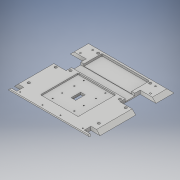
# Autodesk Inventor part: blacha
Saved by Autodesk Inventor 2019 (Build 230136000, 136)
## iProperties
Created: 2019-11-12
Part Number: blacha
Material: Generic
Document SubType Name: Modeling
Designer: Michal
Density: 1 g/cm^3
Appearance: Default
Author: Michal
Autodesk Inventor part; units mm, degrees
ref_plane "YZ Plane" through (0, 0, 0) normal (1, 0, 0) x (0, 1, 0)
ref_plane "XZ Plane" through (0, 0, 0) normal (0, 1, 0) x (-1, 0, 0)
ref_plane "XY Plane" through (0, 0, 0) normal (0, 0, 1) x (1, 0, 0)
sketch "Sketch1" plane through (0, 0, 0) normal (0, 1, 0) x (-1, 0, 0)
  line L0 (0, 0) -> (180, 0)
  line L1 (180, 0) -> (180, -180)
  line L2 (180, -180) -> (0, -180)
  line L3 (0, -180) -> (0, 0)
  line L4 (0, 0) -> (0, -4)
  line L5 (0, -4) -> (15, -4)
  line L6 (15, -4) -> (15, -19)
  line L7 (15, -19) -> (0, -19)
  line L8 (0, -19) -> (0, -4)
  line L9 (90, 0) -> (90, -180)
  line L10 (180, 0) -> (180, -4)
  line L11 (180, -4) -> (165, -4)
  line L12 (165, -4) -> (165, -19)
  line L13 (165, -19) -> (180, -19)
  line L14 (180, -19) -> (180, -4)
  dimension "d0" = 180
  dimension "d1" = 180
  dimension "d2" = 4
  dimension "d3" = 15
  dimension "d4" = 15
  constraints: 30 end point, 4 parallel, 4 symmetric about line, 2 horizontal, 2 midpoint, 2 perpendicular, 1 point on line
  measures "d0" distance of L1.end L2.end
  measures "d1" distance of L0.end L1.end
  measures "d2" distance of L0.start L4.end
  measures "d3" distance of L6.end L7.end
  measures "d4" distance of L5.end L6.end
extrude "Extrusion1" add sketch "Sketch1" along normal blind 8 contours L0 L9 L2 L3 L7 L6 L5 | L0 L1 L11 L12 L13 L2 L9
sketch "Sketch3" plane through (0, 8, 0) normal (0, 1, 0) x (1, 0, 0)
  line L0 (0, 180) -> (-180, 180) projected
  line L1 (0, 180) -> (-30, 180)
  line L2 (-30, 180) -> (-30, 96)
  line L3 (-30, 96) -> (0, 96)
  line L4 (0, 96) -> (0, 180)
  line L5 (-30, 96) -> (-30, 146)
  line L6 (-30, 146) -> (0, 146)
  line L7 (0, 19) -> (0, 180) projected
  line L8 (-30, 96) -> (0, 96)
  line L9 (0, 96) -> (0, 146)
  line L10 (-90, 180) -> (-90, 0)
  line L11 (-180, 180) -> (-150, 180)
  line L12 (-150, 180) -> (-150, 96)
  line L13 (-150, 96) -> (-180, 96)
  line L14 (-180, 96) -> (-180, 180)
  line L15 (-150, 96) -> (-150, 146)
  line L16 (-150, 146) -> (-180, 146)
  line L17 (-150, 96) -> (-180, 96)
  line L18 (-180, 96) -> (-180, 146)
  point P0 (0, 0)
  dimension "d40" = 30
  dimension "d41" = 84
  dimension "d42" = 50
  constraints: 34 end point, 5 symmetric about line, 3 perpendicular, 3 point on line, 2 parallel, 1 collinear, 1 horizontal, 1 midpoint, 1 vertical
  measures "d40" distance of L3.end L2.end
  measures "d41" distance of L2.end L1.end
  measures "d42" distance of L2.end L5.end
extrude "Extrusion2" cut sketch "Sketch3" against normal blind 8 contours L4 L3 L2 L6 | L12 L13 L14 L16
sketch "Sketch4" plane through (0, 0, 0) normal (0, -1, 0) x (1, 0, 0)
  line L0 (0, 0) -> (-180.0098, 0)
  line L1 (-180.0098, 0) -> (-180.0098, -9.1)
  line L2 (-180.0098, -9.1) -> (0, -9.1)
  line L3 (0, -9.1) -> (0, 0)
  dimension "d14" = 180.0098
  dimension "d15" = 9.1
  constraints: 8 end point, 2 parallel, 1 horizontal, 1 perpendicular
  measures "d14" distance of L2.end L1.end
  measures "d15" distance of L1.end L0.end
extrude "Extrusion3" cut sketch "Sketch4" against normal blind 5
sketch "Sketch5" plane through (0, 8, 0) normal (0, 1, 0) x (1, 0, 0)
  line L0 (-0.001, 131.5) -> (-62.0024, 131.5)
  line L1 (-0.001, 110.5) -> (-62.0024, 110.5)
  line L2 (-180.0014, 131.5) -> (-118, 131.5)
  line L3 (-180.0014, 110.5) -> (-118, 110.5)
  line L4 (-62.0024, 110.5) -> (-118, 110.5)
  line L5 (-118, 131.5) -> (-62.0024, 131.5)
  line L6 (-180.0014, 110.5) -> (-180.0014, 131.5)
  line L7 (-0.001, 131.5) -> (-0.001, 110.5)
  line L8 (-150, 146) -> (-150, 96) projected
  line L9 (-150, 150.5) -> (-150, 125.5)
  line L10 (-180.0014, 121) -> (-150, 121)
  point P0 (0, 0)
  point P1 (-61.993, 96)
  point P2 (-118, 96)
  dimension "d19" = 62.0014
  dimension "d21" = 62.0014
  dimension "d47" = 20.5
  constraints: 20 end point, 2 parallel, 1 coincident, 1 horizontal, 1 midpoint, 1 perpendicular, 1 vertical
  measures "d19" distance of L0.end L0.start
  measures "d21" distance of L1.start L1.end
  measures "d47" distance of L8.start L9.end
extrude "Extrusion4" cut sketch "Sketch5" against normal blind 5.5
sketch "Sketch8" plane through (0, 8, 0) normal (0, 1, 0) x (1, 0, 0)
  line L0 (-150, 131.5) -> (-147, 131.5)
  line L1 (-30, 131.5) -> (-33, 131.5)
  line L2 (-40, 131.5) -> (-140, 131.5)
  line L3 (-150, 131.5) -> (-30, 131.5) projected
  line L4 (-150, 131.5) -> (-30, 131.5) projected
  line L5 (-140, 131.5) -> (-137, 131.5)
  line L6 (-137, 171.5) -> (-43, 171.5)
  line L7 (-140, 131.5) -> (-143, 131.5)
  line L8 (-143, 131.5) -> (-143, 171.5)
  line L9 (-43, 131.5) -> (-37, 131.5)
  line L10 (-37, 131.5) -> (-37, 171.5)
  line L11 (-37, 171.5) -> (-143, 171.5)
  point P0 (0, 0)
  dimension "d43" = 3
  dimension "d45" = 3
  dimension "d171" = 3
  dimension "d172" = 3
  dimension "d176" = 3
  dimension "d177" = 6
  constraints: 20 end point, 2 collinear, 2 perpendicular, 5 other
  measures "d43" distance of L0.start L0.end
  measures "d45" distance of L1.start L1.end
  measures "d171" distance of L2.start L9.start
  measures "d172" distance of L2.end L5.end
  measures "d176" distance of L2.end L7.end
  measures "d177" distance of L9.start L9.end
extrude "Extrusion7" cut sketch "Sketch8" against normal blind 4.5
fillet "Fillet1" radius 2 2 edges at (-143, 5.75, -171.5) (-37, 5.75, -171.5)
sketch "Sketch9" plane through (0, 8, 0) normal (0, 1, 0) x (1, 0, 0)
  line L0 (-30, 110.5) -> (-150, 110.5) projected
  line L1 (-90, 110.5) -> (-90, 107.5)
  line L2 (-90, 107.5) -> (-130, 107.5)
  line L3 (-130, 107.5) -> (-130, 27.5)
  line L4 (-130, 27.5) -> (-50, 27.5)
  line L5 (-50, 27.5) -> (-50, 107.5)
  line L6 (-50, 107.5) -> (-90, 107.5)
  point P0 (0, 0)
  dimension "d48" = 3
  dimension "d49" = 40
  dimension "d50" = 80
  dimension "d51" = 80
  constraints: 12 end point, 3 perpendicular, 2 horizontal, 1 midpoint, 1 vertical
  measures "d48" distance of L1.start L1.end
  measures "d49" distance of L1.end L2.end
  measures "d50" distance of L2.end L3.end
  measures "d51" distance of L3.end L4.end
extrude "Extrusion8" cut sketch "Sketch9" against normal blind 3
sketch "Sketch10" plane through (0, 5, 0) normal (0, 1, 0) x (1, 0, 0)
  line L0 (-130, 107.5) -> (-50, 107.5) projected
  line L1 (-130, 107.5) -> (-114.1, 107.5)
  line L2 (-114.1, 107.5) -> (-114.1, 102.1)
  line L3 (-114.1, 102.1) -> (-114.1, 53.9)
  line L4 (-90, 107.5) -> (-90, 27.5)
  line L5 (-50, 27.5) -> (-130, 27.5) projected
  line L6 (-50, 107.5) -> (-65.9, 107.5)
  line L7 (-65.9, 107.5) -> (-65.9, 102.1)
  line L8 (-65.9, 102.1) -> (-65.9, 53.9)
  line L9 (-130, 27.5) -> (-130, 107.5) projected
  line L10 (-130, 67.5) -> (-48.2332, 67.5)
  line L11 (-130, 27.5) -> (-50, 27.5)
  line L12 (-130, 27.5) -> (-114.1, 27.5)
  line L13 (-114.1, 27.5) -> (-114.1, 32.9)
  line L14 (-114.1, 32.9) -> (-114.1, 81.1)
  line L15 (-90, 27.5) -> (-90, 107.5)
  line L16 (-50, 107.5) -> (-130, 107.5)
  line L17 (-50, 27.5) -> (-65.9, 27.5)
  line L18 (-65.9, 27.5) -> (-65.9, 32.9)
  line L19 (-65.9, 32.9) -> (-65.9, 81.1)
  line L20 (-130, 107.5) -> (-130, 27.5)
  point P0 (0, 0)
  dimension "d86" = 15.9
  dimension "d87" = 5.4
  dimension "d88" = 48.2
  constraints: 36 end point, 15 symmetric about line, 3 midpoint, 2 point on line, 2 vertical, 1 perpendicular
  measures "d86" distance of L0.start L1.end
  measures "d87" distance of L1.end L2.end
  measures "d88" distance of L2.end L3.end
move faces "Move1" translate (0, 0, 4) faces at (-103.3333, 7, -27.5)
move faces "Move2" translate (-2, 0, 0) faces at (-130, 6, -79.5)
move faces "Move3" translate (2, 0, 0) faces at (-50, 7, -51.5)
fillet "Fillet2" radius 2 4 edges at (-132, 6.5, -23.5) (-48, 6.5, -23.5) (-48, 6.5, -107.5) (-132, 6.5, -107.5)
sketch "Sketch11" plane through (0, 5, 0) normal (0, -1, 0) x (1, 0, 0)
  line L0 (-165, -9.1) -> (-165, -4) projected
  line L1 (-165, -9.1) -> (-165, -6.1)
  line L2 (-165, -6.1) -> (-160, -6.1)
  line L3 (-160, -6.1) -> (-110, -6.1)
  line L4 (-180, 0) -> (0, 0) projected
  line L5 (-90, 0) -> (-90, -9.1)
  line L6 (-15, -9.1) -> (-165, -9.1) projected
  line L7 (-15, -9.1) -> (-15, -4)
  line L8 (-15, -9.1) -> (-15, -6.1)
  line L9 (-15, -6.1) -> (-20, -6.1)
  line L10 (-20, -6.1) -> (-70, -6.1)
  line L11 (0, 0) -> (-180, 0)
  line L12 (-165, -9.1) -> (-15, -9.1)
  dimension "d64" = 3
  dimension "d65" = 5
  dimension "d66" = 50
  constraints: 20 end point, 8 symmetric about line, 4 point on line, 2 midpoint, 1 perpendicular
  measures "d64" distance of L0.start L1.end
  measures "d65" distance of L1.end L2.end
  measures "d66" distance of L2.end L3.end
hole "Hole1" at (-160, 5, -6.1) at (-110, 5, -6.1) at (-70, 5, -6.1) at (-20, 5, -6.1) direction (0, 1, 0) diameter 2.4638 end through all
move faces "Move4" translate (0, 0, 2.5) faces at (-10, 5.3333, -146)
move faces "Move5" translate (0, 0, 2.5) faces at (-160, 5.3333, -146)
move faces "Move6" translate (0, 0, -2.5) faces at (-160, 2.6667, -96)
move faces "Move7" translate (0, 0, -2.5) faces at (-20, 5.3333, -96)
hole "Hole2" at (-114.1, 5, -102.1) at (-114.1, 5, -53.9) at (-65.9, 5, -53.9) at (-65.9, 5, -102.1) at (-114.1, 5, -81.1) at (-114.1, 5, -32.9) at (-65.9, 5, -32.9) at (-65.9, 5, -81.1) direction (0, -1, 0) diameter 2.4638 end through all
sketch "Sketch15" plane through (0, 0, 0) normal (0, -1, 0) x (1, 0, 0)
  line L0 (0, -180) -> (-180, -180) projected
  line L1 (-180, 0) -> (0, 0) projected
  line L2 (-90, 0) -> (-90, -180)
  line L3 (-149.9592, -180) -> (-149.9592, -168)
  line L4 (-180, -98.5) -> (-150, -98.5)
  line L5 (-149.9592, -168) -> (-159.9592, -168)
  line L6 (-180, -143.5) -> (-150, -143.5)
  line L7 (-180, -143.5) -> (-180, -148.5)
  line L8 (-180, -143.5) -> (-180, -180)
  line L9 (-180, -148.5) -> (-168, -148.5)
  line L10 (-180, -98.5) -> (-168, -98.5)
  line L11 (-150, -98.5) -> (-180, -98.5)
  line L12 (-168, -98.5) -> (-168, -93.5)
  line L13 (-168, -93.5) -> (-168, -33.5)
  line L14 (-149.9592, -168) -> (-147.9592, -168)
  line L15 (-150, -110.5) -> (-150, -98.5) projected
  line L16 (-150, -98.5) -> (-150, -103.5)
  line L17 (-150, -103.5) -> (-145, -103.5)
  line L18 (0, -98.5) -> (-30, -98.5)
  line L19 (-30, -98.5) -> (0, -98.5)
  line L20 (-12, -98.5) -> (-12, -93.5)
  line L21 (-12, -93.5) -> (-12, -33.5)
  line L22 (0, -98.5) -> (-12, -98.5)
  line L23 (0, -143.5) -> (-30, -143.5)
  line L24 (0, -148.5) -> (-12, -148.5)
  line L25 (0, -143.5) -> (0, -148.5)
  line L26 (-30.0408, -168) -> (-20.0408, -168)
  line L27 (0, -143.5) -> (0, -180)
  line L28 (-30.0408, -180) -> (-30.0408, -168)
  line L29 (-30.0408, -168) -> (-32.0408, -168)
  line L30 (-30, -110.5) -> (-30, -98.5)
  line L31 (-30, -98.5) -> (-30, -103.5)
  line L32 (-30, -103.5) -> (-35, -103.5)
  point P0 (-165, -19)
  point P1 (-180, -19)
  point P2 (-15, -19)
  point P3 (0, -19)
  dimension "d173" = 2
  dimension "d174" = 5
  dimension "d175" = 5
  constraints: 60 end point, 18 symmetric about line, 8 point on line, 2 midpoint, 1 horizontal, 1 perpendicular
  measures "d173" distance of L5.start L14.end
  measures "d174" distance of L4.end L16.end
  measures "d175" distance of L16.end L17.end
hole "Hole3" at (-168, 0, -33.5) at (-168, 0, -93.5) at (-145, 0, -103.5) at (-147.9592, 0, -168) at (-12, 0, -33.5) at (-35, 0, -103.5) at (-32.0408, 0, -168) at (-12, 0, -93.5) direction (0, 1, 0) diameter 5.4 end through all countersink diameter 10.3886 countersink angle 90 clearance for "Countersunk Flat Head Screw ISO 2009/7046" size "M5" standard "ISO"
sketch "Sketch16" plane through (0, 0, -180) normal (1, 0, 0) x (0, 0, -1)
  line L0 (0, 0) -> (0, 8) projected
  line L1 (0, 8) -> (3, 8)
  line L2 (3, 8) -> (-11.8412, 22.8412)
  line L3 (-11.8412, 22.8412) -> (-13.9625, 20.7199)
  line L4 (-13.9625, 20.7199) -> (-1.2426, 8)
  line L5 (-36.5, 8) -> (0, 8) projected
  line L6 (0, 6.7574) -> (0, 8)
  line L7 (0, 8) -> (-1.2426, 8)
  line L8 (0, 6.7574) -> (-1.2426, 8)
  point P0 (-180, 0)
  dimension "d133" = 3
  dimension "d134" = 45
  dimension "d135" = 3
  constraints: 14 end point, 2 collinear, 2 perpendicular, 2 point on line, 1 horizontal, 1 vertical
  measures "d133" distance of L0.end L1.end
  measures "d134" angle of L2 L1
  measures "d135" distance of L2.end L3.end
extrude "Extrusion9" cut sketch "Sketch16" against normal blind 180 contours L8 L5 L0
sketch "Sketch17" plane through (-180, 8, 0) normal (0, 0, 1) x (1, 0, 0)
  line L0 (180, 0) -> (180, -8) projected
  line L1 (180, 0) -> (183, 0)
  line L2 (183, 0) -> (173.5168, 9.4832)
  line L3 (173.5168, 9.4832) -> (171.3955, 7.3618)
  line L4 (171.3955, 7.3618) -> (178.7574, 0)
  line L5 (180, 0) -> (0, 0) projected
  line L6 (178.7574, 0) -> (180, 0)
  line L7 (178.7574, 0) -> (180, -1.2426)
  line L8 (180, 0) -> (180, -1.2426)
  line L9 (180, -8) -> (0, -8) projected
  line L10 (90, -8) -> (90, 18.8619)
  line L11 (0, 0) -> (0, -8)
  line L12 (0, 0) -> (-3, 0)
  line L13 (-3, 0) -> (6.4832, 9.4832)
  line L14 (6.4832, 9.4832) -> (8.6045, 7.3618)
  line L15 (8.6045, 7.3618) -> (1.2426, 0)
  line L16 (1.2426, 0) -> (0, 0)
  line L17 (1.2426, 0) -> (0, -1.2426)
  line L18 (0, 0) -> (0, -1.2426)
  dimension "d138" = 3
  dimension "d139" = 13.4112
  dimension "d140" = 45
  dimension "d141" = 3
  constraints: 32 end point, 5 symmetric about line, 4 point on line, 2 collinear, 1 horizontal, 1 midpoint, 1 parallel, 1 perpendicular, 1 vertical
  measures "d138" distance of L0.start L1.end
  measures "d139" distance of L1.end L2.end
  measures "d140" angle of L2 L1
  measures "d141" distance of L2.end L3.end
extrude "Extrusion10" cut sketch "Sketch17" against normal blind 180 contours L0 L7 L5 | L17 L11 L5
sketch "Sketch19" plane through (0, 0, -143.5) normal (1, 0, 0) x (0, 0, -1)
  line L0 (0, 6.7574) -> (36.5, 6.7574) projected
  line L1 (36.5, 0) -> (36.5, 6.7574) projected
  line L2 (36.5, 6.7574) -> (36.5, 0)
  line L3 (36.5, 6.7574) -> (50.6986, 6.7574) construction
  line L4 (36.5, 0) -> (43.2574, 0)
  line L5 (36.5, 6.7574) -> (43.2574, 0)
  point P0 (-143.5, 0)
  constraints: 8 end point, 1 collinear, 1 horizontal, 1 perpendicular
extrude "Extrusion11" add sketch "Sketch19" against normal blind 180
sketch "Sketch20" plane through (-180, 5, 0) normal (0, 0, 1) x (1, 0, 0)
  line L0 (0, 1.7574) -> (1.2426, 3) projected
  line L1 (0, 0) -> (180, 0) projected
  line L2 (0, 1.7574) -> (0, 0)
  line L3 (0, 1.7574) -> (6.1976, 1.7574) construction
  line L4 (0, 0) -> (-1.7574, 0)
  line L5 (0, 1.7574) -> (0, -5) projected
  line L6 (-1.7574, 0) -> (0, 1.7574)
  line L7 (50, 3) -> (130, 3) projected
  line L8 (90, 3) -> (90, -5)
  line L9 (180, 1.7574) -> (178.7574, 3)
  line L10 (180, 1.7574) -> (180, 0)
  line L11 (180, 1.7574) -> (173.8024, 1.7574) construction
  line L12 (180, 0) -> (181.7574, 0)
  line L13 (180, 1.7574) -> (180, -5)
  line L14 (181.7574, 0) -> (180, 1.7574)
  constraints: 22 end point, 5 symmetric about line, 2 horizontal, 1 collinear, 1 midpoint, 1 perpendicular, 1 vertical
extrude "Extrusion12" add sketch "Sketch20" against normal blind 4
sketch "Sketch21" plane through (-15, 0, -19) normal (0, 0, 1) x (1, 0, 0)
  line L0 (15, 6.7574) -> (15, 0) projected
  line L1 (15, 6.7574) -> (15, 0)
  line L2 (15, 6.7574) -> (25.4889, -3.7316)
  line L3 (15, 6.7574) -> (29.8336, 6.7574) construction
  line L4 (15, 0) -> (21.7574, 0)
  line L5 (15, 6.7574) -> (21.7574, 0)
  line L6 (-115, 8) -> (-35, 8) projected
  line L7 (-75, 8) -> (-75, 0)
  line L8 (-165, 6.7574) -> (-165, 0)
  line L9 (-165, 6.7574) -> (-165, 0)
  line L10 (-165, 6.7574) -> (-175.4889, -3.7316)
  line L11 (-165, 6.7574) -> (-179.8336, 6.7574) construction
  line L12 (-165, 0) -> (-171.7574, 0)
  line L13 (-165, 6.7574) -> (-171.7574, 0)
  dimension "d154" = 14.8336
  dimension "d155" = 45
  constraints: 24 end point, 5 symmetric about line, 2 horizontal, 2 point on line, 2 vertical, 1 collinear, 1 equal length, 1 midpoint
  measures "d154" distance of L0.start L2.end
  measures "d155" angle of L2 L3
extrude "Extrusion13" add sketch "Sketch21" against normal blind 170
sketch "Sketch22" plane through (0, 0, -189) normal (-1, 0, 0) x (0, 0, 1)
  line L0 (10.2426, 8) -> (45.5, 8) projected
  line L1 (9, 6.7574) -> (2.2426, 0) projected
  line L2 (10.2426, 8) -> (2.2426, 0)
  line L3 (170, 0) -> (0, 0) projected
  line L4 (2.2426, 0) -> (0, 0)
  line L5 (0, 6.7574) -> (0, 0) projected
  line L6 (0, 0) -> (0, 6.7574)
  line L7 (0, 6.7574) -> (10.2426, 8)
  point P0 (189, 0)
  constraints: 8 end point, 3 collinear
extrude "Extrusion14" cut sketch "Sketch22" along normal mid plane 762
sketch "Sketch23" plane through (0, 8, 0) normal (0, 1, 0) x (1, 0, 0)
  line L0 (-180, 98.5) -> (-180, 143.5) projected
  line L1 (-180, 143.5) -> (-180, 98.5)
  line L2 (-180, 98.5) -> (-186.7574, 98.5)
  line L3 (-186.7574, 19) -> (-186.7574, 186.7574) projected
  line L4 (-186.7574, 143.5) -> (-180, 143.5)
  line L5 (-186.7574, 143.5) -> (-186.7574, 98.5)
  line L6 (0, 98.5) -> (0, 143.5) projected
  line L7 (0, 143.5) -> (6.7574, 143.5)
  line L8 (6.7574, 19) -> (6.7574, 186.7574) projected
  line L9 (6.7574, 98.5) -> (6.7574, 143.5)
  line L10 (6.7574, 98.5) -> (0, 98.5)
  line L11 (0, 98.5) -> (0, 143.5)
  point P0 (0, 0)
  constraints: 16 end point, 4 point on line, 3 collinear, 2 horizontal, 2 perpendicular, 1 parallel
extrude "Extrusion15" cut sketch "Sketch23" against normal blind 762
sketch "Sketch24" plane through (-181.7574, 5, 0) normal (0, 0, 1) x (1, 0, 0)
  line L0 (180.5147, 3) -> (3, 3) projected
  line L1 (180.5147, 3) -> (179.0147, 3)
  line L2 (-5, -5) -> (188.5147, -5) projected
  line L3 (188.5147, -5) -> (187.0147, -5)
  line L4 (187.0147, -5) -> (179.0147, 3)
  line L5 (180.5147, 3) -> (188.5147, -5)
  line L6 (151.7574, 3) -> (31.7574, 3) projected
  line L7 (91.7574, 3) -> (91.7574, -5)
  line L8 (3, 3) -> (4.5, 3)
  line L9 (-5, -5) -> (-3.5, -5)
  line L10 (-3.5, -5) -> (4.5, 3)
  line L11 (3, 3) -> (-5, -5)
  point P0 (181.7574, -5)
  point P1 (1.7574, -5)
  dimension "d162" = 1.5
  dimension "d163" = 1.5
  constraints: 18 end point, 3 point on line, 3 symmetric about line, 1 midpoint, 1 perpendicular
  measures "d162" distance of L0.start L1.end
  measures "d163" distance of L2.end L3.end
extrude "Extrusion16" cut sketch "Sketch24" against normal blind 200 contours L5 L2 L4 L0 | L2 L11 L0 L10
sketch "Sketch25" plane through (-30, 2.5, -131.5) normal (1, 0, 0) x (0, 0, -1)
  line L0 (47.2574, 5.5) -> (45.2574, 5.5)
  line L1 (12, 5.5) -> (47.2574, 5.5) projected
  line L2 (55.2574, -2.5) -> (12, -2.5) projected
  line L3 (55.2574, -2.5) -> (53.2574, -2.5)
  line L4 (53.2574, -2.5) -> (45.2574, 5.5)
  line L5 (47.2574, 5.5) -> (55.2574, -2.5)
  line L6 (45.2574, 5.5) -> (44.2574, 5.5)
  line L7 (44.2574, 5.5) -> (52.2574, -2.5)
  line L8 (53.2574, -2.5) -> (52.2574, -2.5)
  point P0 (-131.5, -2.5)
  dimension "d166" = 2
  dimension "d167" = 2
  dimension "d170" = 1
  constraints: 14 end point, 4 point on line, 1 parallel
  measures "d166" distance of L0.start L0.end
  measures "d167" distance of L2.start L3.end
  measures "d170" distance of L0.end L6.end
extrude "Extrusion17" cut sketch "Sketch25" along normal mid plane 1016
sketch "Sketch26" plane through (0, 0, 0) normal (0, -1, 0) x (1, 0, 0)
  line L0 (-177.2574, 0) -> (-2.7426, 0) construction
  line L1 (-90, 0) -> (-90, -183.7574) construction
  line L2 (-185.2574, -183.7574) -> (5.2574, -183.7574) construction
  line L3 (-150, -143.5) -> (-185.2574, -143.5) construction
  point P0 (0, 0)
  point P1 (-168, -148.5)
  point P2 (-160, -168)
  point P3 (-12, -148.5)
  point P4 (-20, -168)
  dimension "d199" = 78
  dimension "d200" = 5
  dimension "d201" = 70
  dimension "d202" = 24.5
  constraints: 2 end point, 2 midpoint, 2 symmetric about line
  measures "d199" distance from line of L1 point (-168, -148.5)
  measures "d200" distance from line of L3 point (-168, -148.5)
  measures "d201" distance from line of L1 point (-160, -168)
  measures "d202" distance from line of L3 point (-160, -168)
hole "Hole4" at (-20, 0, -168) at (-12, 0, -148.5) at (-168, 0, -148.5) at (-160, 0, -168) direction (0, 1, 0) diameter 3.4 end through all countersink diameter 6.9 countersink angle 81.933 clearance for "Countersunk Flat Head Screw ISO 2009/7046" size "M3" standard "ISO"
sketch "Sketch27" plane through (0, 5, 0) normal (0, 1, 0) x (1, 0, 0)
  line L0 (-50, 23.5) -> (-130, 23.5) projected
  line L1 (-90, 23.5) -> (-90, 107.5)
  line L2 (-130, 107.5) -> (-50, 107.5) projected
  circle A0 centre (-114.1, 53.9) radius 1.2319 projected
  line L3 (-114.1, 53.9) -> (-95.1, 53.9)
  line L4 (-95.1, 53.9) -> (-95.1, 55.9)
  line L5 (-95.1, 55.9) -> (-95.1, 62.9)
  circle A1 centre (-65.9, 53.9) radius 1.2319
  line L6 (-65.9, 53.9) -> (-84.9, 53.9)
  line L7 (-84.9, 53.9) -> (-84.9, 55.9)
  line L8 (-84.9, 55.9) -> (-84.9, 62.9)
  line L9 (-84.9, 62.9) -> (-95.1, 62.9)
  line L10 (-95.1, 53.9) -> (-84.9, 53.9)
  line L11 (-132, 25.5) -> (-132, 105.5) projected
  line L12 (-132, 65.5) -> (-48.3182, 65.5)
  circle A2 centre (-114.1, 77.1) radius 1.2319
  line L13 (-114.1, 77.1) -> (-95.1, 77.1)
  line L14 (-95.1, 77.1) -> (-95.1, 75.1)
  line L15 (-95.1, 75.1) -> (-95.1, 68.1)
  circle A3 centre (-65.9, 77.1) radius 1.2319
  line L16 (-65.9, 77.1) -> (-84.9, 77.1)
  line L17 (-84.9, 77.1) -> (-84.9, 75.1)
  line L18 (-84.9, 75.1) -> (-84.9, 68.1)
  line L19 (-84.9, 68.1) -> (-95.1, 68.1)
  line L20 (-95.1, 77.1) -> (-84.9, 77.1)
  point P0 (0, 0)
  dimension "d185" = 19
  dimension "d186" = 2
  dimension "d187" = 7
  constraints: 36 end point, 12 symmetric about line, 4 point on line, 3 centre point, 3 midpoint, 3 perpendicular, 1 collinear, 1 horizontal, 3 other
  measures "d185" distance of L3.start L3.end
  measures "d186" distance of L3.end L4.end
  measures "d187" distance of L4.end L5.end
extrude "Extrusion18" cut sketch "Sketch27" against normal blind 25.4 contours L10 L4 L5 L9 L1 | L1 L9 L8 L7 L10 | L19 L15 L14 L20 L1 | L1 L20 L17 L18 L19
move faces "Move8" translate (0, 0, 1) faces at (-91.7, 3.3333, -77.1)
move faces "Move9" translate (0, 0, -1) faces at (-88.3, 3.3333, -53.9)
move faces "Move10" translate (0, 0, -9.525) faces at (-91.7, 3.3333, -62.9)
body "Solid1"
